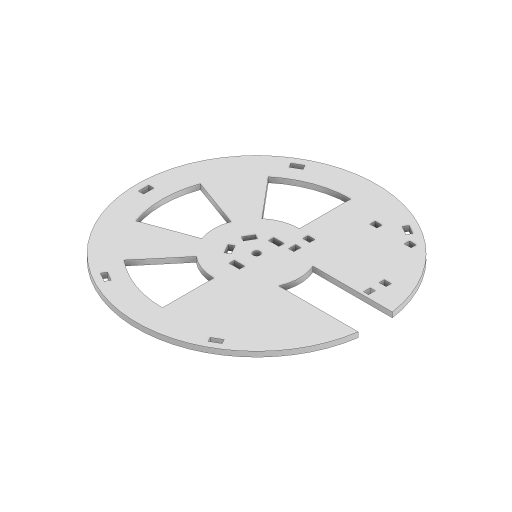
# Autodesk Inventor part: test_circ
Saved by Autodesk Inventor 2024 (Build 280153000, 153)
## iProperties
Created: 2024-04-09
Part Number: test_circ
Material: 一般
Document SubType Name: Modeling
Designer: USER
Density: 1 g/cm^3
Appearance: 預設
Author: USER
Autodesk Inventor part; units mm, degrees
ref_plane "YZ Plane" through (0, 0, 0) normal (1, 0, 0) x (0, 1, 0)
ref_plane "XZ Plane" through (0, 0, 0) normal (0, 1, 0) x (-1, 0, 0)
ref_plane "XY Plane" through (0, 0, 0) normal (0, 0, 1) x (1, 0, 0)
sketch "草圖1" plane through (0, 0, 0) normal (0, 1, 0) x (-1, 0, 0)
  circle A0 centre (0, 0) radius 70
  circle A1 centre (0, 0) radius 25
  line L0 (-70, 10) -> (-10, 10)
  line L1 (-10, 10) -> (-10, -10)
  line L2 (-10, -10) -> (-70, -10)
  line L3 (-70, -10) -> (-70, 10)
  line L4 (0, 0) -> (0, -55)
  line L5 (0, 0) -> (35.3533, -42.1324)
  arc A2 (0, -55) -> (35.3533, -42.1324) centre (0, 0) ccw
  line L6 (0, 0) -> (51.6831, -18.8111)
  line L7 (0, 0) -> (51.6831, 18.8111)
  arc A3 (51.6831, -18.8111) -> (51.6831, 18.8111) centre (0, 0) ccw
  line L8 (0, 0) -> (35.3533, 42.1324)
  line L9 (0, 0) -> (0, 55)
  arc A4 (35.3533, 42.1324) -> (0, 55) centre (0, 0) ccw
  circle A5 centre (0, 0) radius 2
  line L10 (-1.5, 1.3229) -> (-1.5, -1.3229)
  line L11 (-53.6, -11.7755) -> (-50.6, -11.7755)
  line L12 (-10, -11.7968) -> (-7, -11.7968)
  line L13 (-50.6, -11.8181) -> (-50.6, -15.8181)
  line L14 (-50.6, -15.8181) -> (-53.6, -15.8181)
  line L15 (-53.6, -15.8181) -> (-53.6, -11.8181)
  line L16 (-7, -11.7968) -> (-7, -15.7968)
  line L17 (-7, -15.7968) -> (-10, -15.7968)
  line L18 (-10, -15.7968) -> (-10, -11.7968)
  line L19 (-42.3, -47.9058) -> (-38.3, -47.9058)
  line L20 (-38.3, -47.9058) -> (-38.3, -50.9058)
  line L21 (-38.3, -50.9058) -> (-42.3, -50.9058)
  line L22 (-42.3, -50.9058) -> (-42.3, -47.9058)
  line L23 (-22.3, -47.9058) -> (-18.3, -47.9058)
  line L24 (-18.3, -47.9058) -> (-18.3, -50.9058)
  line L25 (-18.3, -50.9058) -> (-22.3, -50.9058)
  line L26 (-22.3, -50.9058) -> (-22.3, -47.9058)
  line L27 (-10, -10) -> (-10, -11.349)
  line L28 (-50.6, -11.8181) -> (-53.6, -11.8181)
  line L29 (-53.6, -11.8181) -> (-53.6, -15.8181)
  line L30 (-50.6, -15.8181) -> (-50.6, -11.8181)
  line L31 (-4, -24) -> (-4, -21) construction
  line L32 (-10, -21) -> (-6, -21) construction
  line L33 (-6, -21) -> (-4, -21) construction
  line L34 (-6, -24) -> (-4, -24) construction
  line L35 (-10, -24) -> (-6, -24) construction
  line L36 (-12, -24) -> (-12, -21) construction
  line L37 (-6, -21) -> (-10, -21)
  line L38 (-10, -21) -> (-10, -24)
  line L39 (-10, -24) -> (-6, -24)
  line L40 (-6, -24) -> (-6, -21)
  line L41 (-50.6, -24) -> (-54.6, -24)
  line L42 (-54.6, -24) -> (-54.6, -21)
  line L43 (-54.6, -21) -> (-50.6, -21)
  line L44 (-50.6, -21) -> (-50.6, -24)
  line L45 (-10, -16.4) -> (-10, -21)
  point P0 (-23, -10)
  point P1 (16.0697, -19.1511)
  point P2 (0, -25)
  point P3 (-69.282, 10)
  point P4 (-69.282, -10)
  point P5 (16.0697, 19.1511)
  point P6 (0, 25)
  point P7 (23.4923, -8.5505)
  point P8 (23.4923, 8.5505)
  point P9 (-70, 0)
  point P10 (-10, 0)
  point P11 (-23, -7)
  point P12 (-52.6, -24)
  point P13 (-8, -24)
  point P14 (-22.9129, 10)
  point P15 (-22.9129, -10)
  dimension "d0" = 140
  dimension "d1" = 50
  dimension "d2" = 20
  dimension "d3" = 60
  dimension "d5" = 40
  dimension "d6" = 55
  dimension "d9" = 140
  dimension "d28" = 4
  dimension "d29" = 1.5
  dimension "d32" = 13
  dimension "d57" = 1.349
  dimension "d58" = 40.6
  dimension "d59" = 4.6
  constraints: 92 end point, 11 equal length, 8 point on circle, 6 coincident, 5 centre point, 5 horizontal, 4 midpoint, 4 point on line, 4 vertical, 3 perpendicular, 2 horizontal alignment, 20 other
  measures "d1" diameter of A1
  measures "d2" distance of L2.end L0.start
  measures "d3" distance of L1.end L2.end
  measures "d5" angle of L4 L5
  measures "d6" distance of L4.start L5.end
  measures "d28" diameter of A5
  measures "d29" distance between parallel lines of L4 L10
  measures "d32" horizontal distance of point (-10, 0) point (-23, -7)
  measures "d57" distance of L1.end L27.end
  measures "d58" distance of L35.start L41.start
  measures "d59" distance of L45.start L45.end
extrude "擠出1" add sketch "草圖1" along normal blind 3 contours A0 L2 A1 L38 L39 L4 A2 L5 L6 A3 L7 L8 A4 L9 L0 | L0 L1 L2 A1 | A1 L9 A5 L4 L39 L40 L37 L38 L2 L1 L0 | A1 L8 A5 L9 | A1 L7 A5 L8 | A1 L6 A5 L7 | L4 A5 L5 A1 | A5 L6 A1 L5
sketch "草圖2" plane through (0, 3, 0) normal (0, 1, 0) x (1, 0, 0)
  line L0 (-3, 13) -> (3, 13)
  line L1 (3, 13) -> (3, 10)
  line L2 (3, 10) -> (-3, 10)
  line L3 (-3, 10) -> (-3, 13)
  line L4 (-12.7583, 3.9019) -> (-9.7583, 9.0981)
  line L5 (-9.7583, 9.0981) -> (-7.1603, 7.5981)
  line L6 (-7.1603, 7.5981) -> (-10.1603, 2.4019)
  line L7 (-10.1603, 2.4019) -> (-12.7583, 3.9019)
  line L8 (-9.7583, -9.0981) -> (-12.7583, -3.9019)
  line L9 (-12.7583, -3.9019) -> (-10.1603, -2.4019)
  line L10 (-10.1603, -2.4019) -> (-7.1603, -7.5981)
  line L11 (-7.1603, -7.5981) -> (-9.7583, -9.0981)
  line L12 (3, -13) -> (-3, -13)
  line L13 (-3, -13) -> (-3, -10)
  line L14 (-3, -10) -> (3, -10)
  line L15 (3, -10) -> (3, -13)
  line L16 (-66, 3) -> (-63, 3)
  line L17 (-63, 3) -> (-63, -3)
  line L18 (-63, -3) -> (-66, -3)
  line L19 (-66, -3) -> (-66, 3)
  line L20 (-34.0981, -53.0596) -> (-28.9019, -56.0596)
  line L21 (-28.9019, -56.0596) -> (-30.4019, -58.6577)
  line L22 (-30.4019, -58.6577) -> (-35.5981, -55.6577)
  line L23 (-35.5981, -55.6577) -> (-34.0981, -53.0596)
  line L24 (28.9019, -56.0596) -> (34.0981, -53.0596)
  line L25 (34.0981, -53.0596) -> (35.5981, -55.6577)
  line L26 (35.5981, -55.6577) -> (30.4019, -58.6577)
  line L27 (30.4019, -58.6577) -> (28.9019, -56.0596)
  line L28 (63, -3) -> (63, 3)
  line L29 (63, 3) -> (66, 3)
  line L30 (66, 3) -> (66, -3)
  line L31 (66, -3) -> (63, -3)
  line L32 (34.0981, 53.0596) -> (28.9019, 56.0596)
  line L33 (28.9019, 56.0596) -> (30.4019, 58.6577)
  line L34 (30.4019, 58.6577) -> (35.5981, 55.6577)
  line L35 (35.5981, 55.6577) -> (34.0981, 53.0596)
  line L36 (-28.9019, 56.0596) -> (-34.0981, 53.0596)
  line L37 (-34.0981, 53.0596) -> (-35.5981, 55.6577)
  line L38 (-35.5981, 55.6577) -> (-30.4019, 58.6577)
  line L39 (-30.4019, 58.6577) -> (-28.9019, 56.0596)
  point P0 (0, 0)
  point P1 (0, 10)
  point P2 (-8.6603, 5)
  point P3 (-8.6603, -5)
  point P4 (0, -10)
  point P5 (-63, 0)
  point P6 (-31.5, -54.5596)
  point P7 (31.5, -54.5596)
  point P8 (63, 0)
  point P9 (31.5, 54.5596)
  point P10 (-31.5, 54.5596)
  dimension "d33" = 3
  dimension "d34" = 6
  dimension "d35" = 10
  dimension "d38" = 180
  dimension "d49" = 3
  dimension "d50" = 6
  dimension "d51" = 63
  dimension "d54" = 360
  constraints: 80 end point, 4 parallel, 2 horizontal, 2 midpoint, 2 perpendicular, 1 horizontal alignment, 1 vertical alignment, 83 other
  measures "d33" distance of L0.end L1.end
  measures "d34" distance of L1.end L2.end
  measures "d35" distance from line of point (0, 0) L2
  measures "d49" distance of L17.end L18.end
  measures "d50" distance of L16.end L17.end
  measures "d51" distance from line of point (0, 0) L17
extrude "擠出2" cut sketch "草圖2" against normal through all contours L0 L1 L2 L3 | L4 L5 L6 L7 | L8 L9 L10 L11 | L12 L13 L14 L15 | L16 L17 L18 L19 | L20 L21 L22 L23 | L24 L25 L26 L27 | L32 L33 L34 L35 | L36 L37 L38 L39
